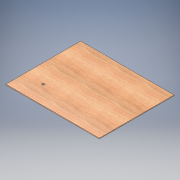
# Autodesk Inventor part: ShooterBaseV02
Saved by Autodesk Inventor 2019.4 (Build 234330000, 330)
## iProperties
Created: 2015-07-21
Part Number: ShooterBaseV02
Material: Wood (Birch)
Document SubType Name: Modeling
Designer: steele
Density: 0.55 g/cm^3
Appearance: Birch - Natural Polished
Mass: 2597.87 g
Surface Area: 10546.3 cm^2
Volume: 4723.41 cm^3
Author: steele
Autodesk Inventor part; units mm, degrees
ref_plane "YZ Plane" through (0, 0, 0) normal (1, 0, 0) x (0, 1, 0)
ref_plane "XZ Plane" through (0, 0, 0) normal (0, 1, 0) x (-1, 0, 0)
ref_plane "XY Plane" through (0, 0, 0) normal (0, 0, 1) x (1, 0, 0)
sketch "Sketch1" plane through (0, 0, 0) normal (0, 1, 0) x (-1, 0, 0)
  line L0 (-381, 304.8) -> (-381, -304.8)
  line L1 (-381, -304.8) -> (381, -304.8)
  line L2 (381, -304.8) -> (381, 304.8)
  line L3 (381, 304.8) -> (-381, 304.8)
  line L4 (-381, 304.8) -> (381, -304.8) construction
  line L5 (-381, -304.8) -> (381, 304.8) construction
  point P0 (0, 0)
  dimension "width" = 609.6
  dimension "length" = 762
  constraints: 12 end point, 2 midpoint, 2 parallel, 1 perpendicular, 1 vertical
  measures "width" distance of L0.start L0.end
  measures "length" distance of L2.end L0.start
extrude "Extrusion1" add sketch "Sketch1" against normal blind 6.35
sketch "Sketch9" plane through (0, 0, 0) normal (0, 1, 0) x (1, 0, 0)
  circle A0 centre (-228.6, -152.4) radius 10.165
  line L0 (-381, -304.8) -> (381, -304.8) projected
  line L1 (-381, 304.8) -> (-381, -304.8) projected
  point P0 (0, 0)
  point P1 (374.65, -304.8)
  point P2 (-381, 298.45)
  dimension "d38" = 152.4
  dimension "d39" = 152.4
  constraints: 1 centre point
  measures "d38" distance from line of A0.centre L0
  measures "d39" distance from line of A0.centre L1
extrude "Extrusion3" cut sketch "Sketch9" against normal through all
body "Solid1"
